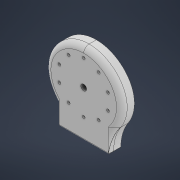
# Autodesk Inventor part: 03_DoF1_Bark
Saved by Autodesk Inventor 2022 (Build 260153000, 153)
## iProperties
Created: 2022-05-07
Part Number: 03_DoF1_Bark
Material: Generic
Document SubType Name: Modeling
Designer: pzach
Density: 1 g/cm^3
Appearance: Default
Author: pzach
Autodesk Inventor part; units mm, degrees
ref_plane "YZ Plane" through (0, 0, 0) normal (1, 0, 0) x (0, 1, 0)
ref_plane "XZ Plane" through (0, 0, 0) normal (0, 1, 0) x (-1, 0, 0)
ref_plane "XY Plane" through (0, 0, 0) normal (0, 0, 1) x (1, 0, 0)
sketch "Sketch1" plane through (0, 0, 0) normal (0, 0, 1) x (1, 0, 0)
  line L0 (0, 0) -> (-391.441, 0)
  line L1 (0, 0) -> (391.441, 0)
  line L2 (391.441, 0) -> (391.441, 250)
  line L3 (391.441, 250) -> (880.679, 727.5784) construction
  line L4 (880.679, 727.5784) -> (510.0425, 1285.2027) construction
  line L5 (510.0425, 1285.2027) -> (99.3373, 1285.2027) construction
  line L6 (99.3373, 1285.2027) -> (0, 1285.2027) construction
  spline S0 degree 4 poles (391.441, 250) (880.679, 727.5784) (510.0425, 1285.2027) (99.3373, 1285.2027) (0, 1285.2027) knots 1 1 1 1 1 2 2 2 2 2
  line L7 (0, 1285.2027) -> (0, 0) construction
  line L8 (-391.441, 0) -> (-391.441, 250)
  line L9 (-391.441, 250) -> (-880.679, 727.5784) construction
  line L10 (-880.679, 727.5784) -> (-510.0425, 1285.2027) construction
  line L11 (-510.0425, 1285.2027) -> (-99.3373, 1285.2027) construction
  line L12 (-99.3373, 1285.2027) -> (0, 1285.2027) construction
  spline S1 degree 4 poles (-391.441, 250) (-880.679, 727.5784) (-510.0425, 1285.2027) (-99.3373, 1285.2027) (0, 1285.2027) knots 1 1 1 1 1 2 2 2 2 2
  line L13 (0, 0) -> (0, 1285.2027) construction
  line L14 (0, 1285.2027) -> (0, 1135.2027) construction
  point P0 (0, 727.5784)
  dimension "d1" = 391.441
  dimension "d2" = 250
  dimension "d15" = 489.238
  dimension "d16" = 370.6365
  dimension "d17" = 410.7053
  dimension "d18" = 100.698
  dimension "d19" = 123.611
  dimension "d20" = 99.3373
  dimension "d21" = 56.389
  dimension "d24" = 727.5784
  dimension "d32" = 150
  constraints: 14 end point, 4 symmetric about line, 3 point on line, 2 equal length, 2 horizontal, 1 coincident, 1 vertical, 6 other
  measures "d1" distance of L0.start L1.end
  measures "d2" distance of L1.end L2.end
  measures "d15" horizontal distance of L2.end L3.end
  measures "d16" horizontal distance of L3.end L4.end
  measures "d17" distance of L4.end L5.end
  measures "d18" angle of L4 L3
  measures "d19" angle of L5 L4
  measures "d20" distance of L5.end L6.end
  measures "d21" angle of L6 L4
  measures "d24" distance of L0.start point (0, 727.578)
  measures "d32" distance of L6.end L14.end
extrude "Extrusion1" add sketch "Sketch1" along normal blind 200
fillet "Fillet1" radius 85 2 edges at (460.7351, 1081.0964, 200) (-460.7351, 1081.0964, 200)
fillet "Fillet2" radius 20 1 edges at (0, 0, 200)
fillet "Fillet4" radius 705.75 2 edges at (391.441, 250, 57.5) (391.441, 302.8436, 185.1836)
hole "Hole1" at (0, 727.5784, 0) direction (0, 0, 1) diameter 93.505 end through all thread size "M100x6" class "6H" standard "ANSI Metric M Profile"
hole "Hole2" at (0, 1135.2027, 0) direction (0, 0, 1) diameter 45.6699 end through all thread size "M50x4" class "6H" standard "ANSI Metric M Profile"
pattern_circular "Circular Pattern1" count 10 over 360 about axis through (0, 727.5784, 2189.5561) along (0, 0, 1) of "Hole2"
equation "\"d1\" = d0"
equation "\"d0\" = 391.441"
body "Solid1"
